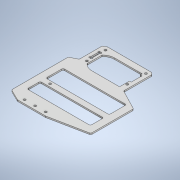
# Autodesk Inventor part: Trunk_upper_flank_frame
Saved by Autodesk Inventor 2020.4 (Build 244396000, 396)
## iProperties
Created: 2021-09-10
Part Number: Trunk_upper_flank_frame
Material: GFRP
Document SubType Name: Modeling
Designer: Masato Kubotera
Density: 1.75 g/cm^3
Appearance: 滑らか - 淡い灰色
Description: GFRP T2
Mass: 17.4509 g
Surface Area: 121.173 cm^2
Volume: 9.97196 cm^3
Author: Masato Kubotera
Autodesk Inventor part; units mm, degrees
ref_plane "YZ Plane" through (0, 0, 0) normal (1, 0, 0) x (0, 1, 0)
ref_plane "XZ Plane" through (0, 0, 0) normal (0, 1, 0) x (-1, 0, 0)
ref_plane "XY Plane" through (0, 0, 0) normal (0, 0, 1) x (1, 0, 0)
sketch "スケッチ1" plane through (0, 0, 0) normal (0, 0, 1) x (1, 0, 0)
  circle A0 centre (0, 0) radius 11
  line L0 (-0.3073, 13.5) -> (26.6927, 13.5) construction
  line L1 (26.6927, 13.5) -> (26.6927, -13.5) construction
  line L2 (26.6927, -13.5) -> (-0.3073, -13.5) construction
  line L3 (-0.3073, -13.5) -> (-0.3073, 13.5) construction
  line L4 (-0.3073, 13.5) -> (26.6927, -13.5) construction
  line L5 (26.6927, 13.5) -> (-0.3073, -13.5) construction
  line L6 (-12, 16) -> (39.5, 16) construction
  line L7 (39.5, 16) -> (39.5, -16) construction
  line L8 (39.5, -16) -> (-12, -16) construction
  line L9 (-12, -16) -> (-12, 16) construction
  line L10 (-12, 16) -> (39.5, -16) construction
  line L11 (39.5, 16) -> (-12, -16) construction
  circle A1 centre (-0.3073, 13.5) radius 1.35
  arc A2 (0, 16) -> (-12, 10.583) centre (0, 0) ccw construction
  line L12 (-12, 0) -> (39.5, 0)
  circle A3 centre (26.6927, 13.5) radius 1.35
  arc A4 (-12, -10.583) -> (0, -16) centre (0, 0) ccw construction
  circle A5 centre (-0.3073, -13.5) radius 1.35
  circle A6 centre (26.6927, -13.5) radius 1.35
  arc A7 (0, 16.05) -> (-12.05, 10.6019) centre (0, 0) ccw
  line L13 (0, 16.05) -> (39.55, 16.05)
  line L14 (39.55, 16.05) -> (39.55, 13.3)
  line L15 (-12.05, 10.6019) -> (-12.05, 0)
  arc A8 (-11.5146, 11.1811) -> (-12.05, 9.86) centre (-11.0677, 10.2309) ccw
  line L16 (-12.05, 10.6019) -> (-11.0677, 10.2309) construction
  arc A9 (39.55, 14.5651) -> (38.0651, 16.05) centre (38.8075, 15.3075) ccw
  line L17 (38.8075, 15.3075) -> (39.55, 16.05) construction
  arc A10 (-12.05, -10.6019) -> (0, -16.05) centre (0, 0) ccw
  line L18 (0, -16.05) -> (39.55, -16.05)
  line L19 (-12.05, -10.6019) -> (-12.05, 0)
  arc A11 (-12.05, -9.86) -> (-11.5146, -11.1811) centre (-11.0677, -10.2309) ccw
  arc A12 (38.0651, -16.05) -> (39.55, -14.5651) centre (38.8075, -15.3075) ccw
  line L20 (39.55, 13.3) -> (42.05, 13.3)
  line L21 (42.05, 13.3) -> (42.05, -1.8)
  line L22 (42.05, -1.8) -> (39.55, -1.8)
  line L23 (39.55, -1.8) -> (39.55, -14.5651)
  line L24 (39.5, 13.25) -> (42, 13.25) construction
  line L25 (42, 13.25) -> (42, -1.75) construction
  line L26 (42, -1.75) -> (39.5, -1.75) construction
  line L27 (42, 5.75) -> (39.5, 5.75) construction
  arc A13 (42.05, 11.8151) -> (40.5651, 13.3) centre (41.3075, 12.5575) ccw
  line L28 (41.3075, 12.5575) -> (42.05, 13.3) construction
  arc A14 (40.5651, -1.8) -> (42.05, -0.3151) centre (41.3075, -1.0575) ccw
  circle A15 centre (-15.5, 19) radius 1.6
  line L29 (-18, 22) -> (-13, 22) construction
  line L30 (-13, 22) -> (-13, -10.5) construction
  line L31 (-13, -10.5) -> (-18, -10.5) construction
  line L32 (-18, -10.5) -> (-18, 22) construction
  line L33 (-18, 22) -> (-13, -10.5) construction
  line L34 (-13, 22) -> (-18, -10.5) construction
  line L35 (-18, 5.75) -> (-13, 5.75) construction
  line L36 (-15.5, 22) -> (-15.5, -10.5) construction
  line L37 (-18, 13.25) -> (-15.5, 13.25) construction
  line L38 (-15.5, 13.25) -> (-15.5, -1.75) construction
  line L39 (-15.5, -1.75) -> (-18, -1.75) construction
  line L40 (-18, 13.25) -> (-15.5, -1.75) construction
  line L41 (-15.5, 13.25) -> (-18, -1.75) construction
  line L42 (-15.45, -1.8) -> (-18.05, -1.8)
  line L43 (-18.05, -1.8) -> (-18.05, 13.3)
  line L44 (-18.05, 13.3) -> (-15.45, 13.3)
  line L45 (-15.45, 13.3) -> (-15.45, -1.8)
  line L46 (-15.45, -1.8) -> (-18.05, 13.3) construction
  line L47 (-18.05, -1.8) -> (-15.45, 13.3) construction
  line L48 (-16.75, 13.3) -> (-16.75, -1.8) construction
  arc A16 (-18.05, 13.3) -> (-18.05, 11.2) centre (-18.05, 12.25) ccw
  arc A17 (-15.45, 11.2) -> (-15.45, 13.3) centre (-15.45, 12.25) ccw
  arc A18 (-18.05, 0.3) -> (-18.05, -1.8) centre (-18.05, -0.75) ccw
  arc A19 (-15.45, -1.8) -> (-15.45, 0.3) centre (-15.45, -0.75) ccw
  circle A20 centre (-15.5, -7.5) radius 1.6
  line L49 (13.1927, 16) -> (13.1927, -16) construction
  circle A21 centre (42, 19) radius 1.6
  line L50 (39.5, 22) -> (44.5, 22) construction
  line L51 (44.5, 22) -> (44.5, -10.5) construction
  line L52 (44.5, -10.5) -> (39.5, -10.5) construction
  line L53 (39.5, 22) -> (44.5, -10.5) construction
  line L54 (44.5, 22) -> (39.5, -10.5) construction
  line L55 (42, 22) -> (42, -10.5) construction
  circle A22 centre (42, -7.5) radius 1.6
  line L56 (-12, 23.25) -> (-12, 18.25) construction
  line L57 (-18, 24.5) -> (44.5, 24.5)
  line L58 (-18, 24.5) -> (-23, 22)
  line L59 (44.5, 24.5) -> (47.5, 22)
  line L60 (-23, 22) -> (-23, -10.75)
  line L61 (47.5, 22) -> (47.5, -18.25)
  line L62 (47.5, -18.25) -> (76.5, -33.25)
  line L63 (-23, -10.75) -> (-33.5, -16)
  line L64 (-33.5, -16) -> (-33.5, -96.5)
  line L65 (76.5, -33.25) -> (76.5, -93.8101)
  line L66 (76.5, -93.8101) -> (23, -104.5)
  line L67 (23, -104.5) -> (-17, -104.5)
  line L68 (-17, -104.5) -> (-33.5, -96.5)
  circle A23 centre (-12, -99.5) radius 1.6
  circle A24 centre (3, -99.5) radius 1.6
  line L69 (-17, -104.5) -> (-17, -94.5) construction
  line L70 (-17, -94.5) -> (23, -94.5) construction
  line L71 (23, -94.5) -> (23, -104.5) construction
  line L72 (-17, -99.5) -> (23, -99.5) construction
  line L73 (3, -94.5) -> (3, -104.5) construction
  circle A25 centre (18, -99.5) radius 1.6
  circle A26 centre (-13.5, -61.75) radius 1.6
  line L74 (-23.5, -65.75) -> (66.5, -65.75)
  line L75 (66.5, -65.75) -> (66.5, -84.5)
  line L76 (66.5, -84.5) -> (-23.5, -84.5)
  line L77 (-23.5, -84.5) -> (-23.5, -65.75)
  line L78 (-23.5, -33.25) -> (66.5, -33.25)
  line L79 (66.5, -33.25) -> (66.5, -57.75)
  line L80 (66.5, -57.75) -> (-23.5, -57.75)
  line L81 (-23.5, -57.75) -> (-23.5, -33.25)
  circle A27 centre (-13.5, -61.75) radius 4 construction
  line L82 (-9.8584, -97.6093) -> (-9.2918, -98.5907)
  line L83 (-9.2918, -100.4093) -> (-9.8584, -101.3907)
  line L84 (-11.4334, -102.3) -> (-12.5666, -102.3)
  line L85 (-14.1416, -101.3907) -> (-14.7082, -100.4093)
  line L86 (-14.7082, -98.5907) -> (-14.1416, -97.6093)
  line L87 (-12.5666, -96.7) -> (-11.4334, -96.7)
  arc A28 (-9.8584, -97.6093) -> (-11.4334, -96.7) centre (-10.9084, -97.6093) ccw
  arc A29 (-12.5666, -96.7) -> (-14.1416, -97.6093) centre (-13.0916, -97.6093) ccw
  arc A30 (-14.7082, -98.5907) -> (-14.7082, -100.4093) centre (-14.1832, -99.5) ccw
  arc A31 (-14.1416, -101.3907) -> (-12.5666, -102.3) centre (-13.0916, -101.3907) ccw
  arc A32 (-11.4334, -102.3) -> (-9.8584, -101.3907) centre (-10.9084, -101.3907) ccw
  arc A33 (-9.2918, -100.4093) -> (-9.2918, -98.5907) centre (-9.8168, -99.5) ccw
  arc A34 (5.7082, -100.4093) -> (5.7082, -98.5907) centre (5.1832, -99.5) ccw
  line L88 (5.1416, -97.6093) -> (5.7082, -98.5907)
  line L89 (5.7082, -100.4093) -> (5.1416, -101.3907)
  arc A35 (3.5666, -102.3) -> (5.1416, -101.3907) centre (4.0916, -101.3907) ccw
  arc A36 (5.1416, -97.6093) -> (3.5666, -96.7) centre (4.0916, -97.6093) ccw
  line L90 (2.4334, -96.7) -> (3.5666, -96.7)
  arc A37 (2.4334, -96.7) -> (0.8584, -97.6093) centre (1.9084, -97.6093) ccw
  line L91 (0.2918, -98.5907) -> (0.8584, -97.6093)
  arc A38 (0.2918, -98.5907) -> (0.2918, -100.4093) centre (0.8168, -99.5) ccw
  line L92 (0.8584, -101.3907) -> (0.2918, -100.4093)
  arc A39 (0.8584, -101.3907) -> (2.4334, -102.3) centre (1.9084, -101.3907) ccw
  line L93 (3.5666, -102.3) -> (2.4334, -102.3)
  arc A40 (20.7082, -100.4093) -> (20.7082, -98.5907) centre (20.1832, -99.5) ccw
  line L94 (20.1416, -97.6093) -> (20.7082, -98.5907)
  line L95 (20.7082, -100.4093) -> (20.1416, -101.3907)
  arc A41 (18.5666, -102.3) -> (20.1416, -101.3907) centre (19.0916, -101.3907) ccw
  arc A42 (20.1416, -97.6093) -> (18.5666, -96.7) centre (19.0916, -97.6093) ccw
  line L96 (17.4334, -96.7) -> (18.5666, -96.7)
  arc A43 (17.4334, -96.7) -> (15.8584, -97.6093) centre (16.9084, -97.6093) ccw
  line L97 (15.2918, -98.5907) -> (15.8584, -97.6093)
  arc A44 (15.2918, -98.5907) -> (15.2918, -100.4093) centre (15.8168, -99.5) ccw
  line L98 (15.8584, -101.3907) -> (15.2918, -100.4093)
  arc A45 (15.8584, -101.3907) -> (17.4334, -102.3) centre (16.9084, -101.3907) ccw
  line L99 (18.5666, -102.3) -> (17.4334, -102.3)
  point P0 (13.1927, 0)
  point P1 (-15.5, 5.75)
  point P2 (-16.75, 5.75)
  point P3 (13.1927, 0)
  point P4 (42, 5.75)
  point P5 (42, 5.75)
  point P6 (-18.05, 0.3)
  point P7 (-15.45, 0.3)
  point P8 (42.05, -0.3151)
  point P9 (40.5651, -1.8)
  point P10 (-10.3834, -96.7)
  point P11 (-13.6166, -96.7)
  point P12 (-15.2332, -99.5)
  point P13 (-13.6166, -102.3)
  point P14 (-10.3834, -102.3)
  point P15 (-8.7668, -99.5)
  point P16 (-13.6166, -96.7)
  point P17 (-15.2332, -99.5)
  point P18 (-8.7668, -99.5)
  point P19 (3, -99.5)
  point P20 (6.2332, -99.5)
  point P21 (6.2332, -99.5)
  point P22 (4.6166, -96.7)
  point P23 (4.6166, -102.3)
  point P24 (3, -99.5)
  point P25 (3, -99.5)
  point P26 (1.3834, -96.7)
  point P27 (1.3834, -96.7)
  point P28 (-0.2332, -99.5)
  point P29 (-0.2332, -99.5)
  point P30 (1.3834, -102.3)
  point P31 (18, -99.5)
  point P32 (21.2332, -99.5)
  point P33 (21.2332, -99.5)
  point P34 (19.6166, -96.7)
  point P35 (19.6166, -102.3)
  point P36 (18, -99.5)
  point P37 (18, -99.5)
  point P38 (16.3834, -96.7)
  point P39 (16.3834, -96.7)
  point P40 (14.7668, -99.5)
  point P41 (14.7668, -99.5)
  point P42 (16.3834, -102.3)
  dimension "d0" = 22
  dimension "d1" = 27
  dimension "d2" = 27
  dimension "d5" = 32
  dimension "d8" = 2.7
  dimension "d9" = 16
  dimension "d10" = 2.7
  dimension "d13" = 12
  dimension "d16" = 0.05
  dimension "d17" = 1.05
  dimension "d18" = 0.05
  dimension "d19" = 1.05
  dimension "d21" = 15
  dimension "d23" = 0.05
  dimension "d24" = 0.05
  dimension "d25" = 0.05
  dimension "d26" = 1.05
  dimension "d27" = 3.2
  dimension "d28" = 5
  dimension "d29" = 2.5
  dimension "d30" = 15
  dimension "d32" = 2.6
  dimension "d33" = 15.1
  dimension "d34" = 1.05
  dimension "d35" = 26.5
  dimension "d36" = 5.5
  dimension "d37" = 2.5
  dimension "d38" = 3.2
  dimension "d39" = 5
  dimension "d40" = 32.5
  dimension "d41" = 26.5
  dimension "d55" = 5
  dimension "d56" = 3
  dimension "d57" = 20.5
  dimension "d60" = 40
  dimension "d61" = 8
  dimension "d63" = 3.2
  dimension "d64" = 3.2
  dimension "d66" = 10
  dimension "d70" = 30
  dimension "d71" = 3.2
  dimension "d72" = 32.75
  dimension "d73" = 20
  dimension "d74" = 8
  dimension "d75" = 10
  dimension "d77" = 10
  dimension "d78" = 10
  dimension "d87" = 1.05
  dimension "d88" = 360
  dimension "d89" = 5.6
  dimension "d92" = 15
  dimension "d97" = 120.5
  dimension "d98" = 1
  dimension "d100" = 110
  dimension "d101" = 2.5
  constraints: 200 end point, 74 point on circle, 46 centre point, 44 point on line, 29 midpoint, 25 symmetric about line, 18 perpendicular, 17 parallel, 16 coincident, 12 horizontal, 5 vertical, 3 tangent, 2 collinear, 137 other
  measures "d0" diameter of A0
  measures "d1" distance of L1.end L2.end
  measures "d2" distance of L0.end L1.end
  measures "d5" distance of L6.end L7.end
  measures "d8" diameter of A1
  measures "d9" radius of A2
  measures "d10" diameter of A3
  measures "d13" distance of L12.start point (0, 0)
  measures "d16" distance from line of L15.start L9
  measures "d17" radius of A8
  measures "d18" distance between parallel lines of L7 L14
  measures "d19" radius of A9
  measures "d21" distance of L24.end L25.end
  measures "d23" horizontal distance of L21.end L25.end
  measures "d24" horizontal distance of L21.end L25.end
  measures "d25" horizontal distance of L24.end L20.end
  measures "d26" radius of A13
  measures "d27" diameter of A15
  measures "d28" distance of L30.end L31.end
  measures "d29" distance of L38.end L39.end
  measures "d30" distance of L37.end L38.end
  measures "d32" distance of L43.end L44.end
  measures "d33" distance of L42.end L43.end
  measures "d34" radius of A16
  measures "d35" distance of A20.centre A15.centre
  measures "d36" vertical distance of L30.end L8.end
  measures "d37" distance of L27.start L27.end
  measures "d38" diameter of A21
  measures "d39" distance of L51.end L52.end
  measures "d40" distance of L50.end L51.end
  measures "d41" distance of A22.centre A21.centre
  measures "d55" distance of L58.end L29.start
  measures "d56" distance of L59.end L50.end
  measures "d57" distance from line of L30 L63.end
  measures "d60" distance of L67.end L66.end
  measures "d61" vertical distance of L67.end L64.end
  measures "d63" diameter of A23
  measures "d64" diameter of A24
  measures "d66" distance from line of L70 L67.end
  measures "d70" distance of A25.centre A23.centre
  measures "d71" diameter of A26
  measures "d72" vertical distance of L69.end A26.centre
  measures "d73" distance from line of A26.centre L64
  measures "d74" diameter of A27
  measures "d75" vertical distance of L69.end L76.end
  measures "d77" horizontal distance of L63.end L78.start
  measures "d78" distance of L62.end L78.end
  measures "d87" radius of A28
  measures "d89" distance between parallel lines of L83 L86
  measures "d92" distance of A23.centre point (3, -99.5)
  measures "d97" vertical distance of L67.end L6.start
  measures "d98" distance from line of L29.end L9
  measures "d100" distance between parallel lines of L64 L65
  measures "d101" distance between parallel lines of L57 L29
extrude "押し出し1" add sketch "スケッチ1" along normal blind 2 contours L57 L59 L61 L62 L65 L66 L67 L68 L64 L63 L60 L58 | L82 A33 L83 A32 L84 A31 L85 A30 L86 A29 L87 A28 | L89 A35 L93 A39 L92 A38 L91 A37 L90 A36 L88 A34 | L95 A41 L99 A45 L98 A44 L97 A43 L96 A42 L94 A40
fillet "フィレット1" radius 2 12 edges at (-17, -104.5, 1) (-33.5, -96.5, 1) (-33.5, -16, 1) (-23, -10.75, 1) (23, -104.5, 1) (76.5, -93.8101, 1) (76.5, -33.25, 1) (47.5, -18.25, 1) (47.5, 22, 1) (44.5, 24.5, 1) (-23, 22, 1) (-18, 24.5, 1)
fillet "フィレット2" radius 2 8 edges at (-23.5, -33.25, 1) (-23.5, -57.75, 1) (66.5, -57.75, 1) (66.5, -33.25, 1) (-23.5, -84.5, 1) (-23.5, -65.75, 1) (66.5, -84.5, 1) (66.5, -65.75, 1)
equation "\"d10\" = d8"
equation "\"d16\" = d15"
equation "\"d18\" = d15"
equation "\"d19\" = d17"
equation "\"d23\" = d15"
equation "\"d24\" = d23"
equation "\"d25\" = d15"
equation "\"d26\" = d17"
equation "\"d15\" = 0.05"
